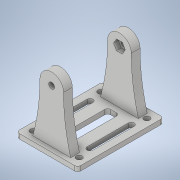
# Autodesk Inventor part: sideArmsHolder
Saved by Autodesk Inventor 2020 (Build 240168000, 168)
## iProperties
Created: 2019-05-25
Part Number: sideArmsHolder
Material: Generic
Document SubType Name: Modeling
Designer: Ryland Lillibridge
Density: 1 g/cm^3
Appearance: Default
Author: Ryland Lillibridge
Autodesk Inventor part; units mm, degrees
ref_plane "YZ Plane" through (0, 0, 0) normal (1, 0, 0) x (0, 1, 0)
ref_plane "XZ Plane" through (0, 0, 0) normal (0, 1, 0) x (-1, 0, 0)
ref_plane "XY Plane" through (0, 0, 0) normal (0, 0, 1) x (1, 0, 0)
sketch "Sketch1" plane through (0, 0, 0) normal (0, 1, 0) x (-1, 0, 0)
  circle A0 centre (0, 0) radius 31.75
  circle A1 centre (0, 0) radius 12.3825
  dimension "d0" = 63.5
  dimension "d1" = 24.765
  constraints: 2 centre point, 2 coincident
  measures "d0" diameter of A0
  measures "d1" diameter of A1
extrude "Extrusion1" add sketch "Sketch1" along normal blind 3.175 contours A0 | A1
sketch "Sketch2" plane through (0, 0, 0) normal (0, -1, 0) x (1, 0, 0)
  line L0 (1.524, 31.713403) -> (1.524, 0)
  line L1 (-1.524, 0) -> (-1.524, 31.713403)
  line L2 (-1.524, 35.89292) -> (0, 0) construction
  line L3 (1.524, 35.89292) -> (0, 0) construction
  line L4 (-1.524, 0) -> (1.524, 0)
  circle A0 centre (0, 0) radius 31.75
  dimension "d23" = 3.048
  constraints: 10 end point, 2 point on circle, 2 point on line, 1 parallel
  measures "d23" distance between parallel lines of L0 L1
extrude "Extrusion2" add sketch "Sketch2" along normal blind 1.524 contours L0 L4 L1 A0 picked at (0.169391, 10.581978)
pattern_circular "Circular Pattern1" count 8 over 360 about axis through (0, -10, 0) along (0, 1, 0) of "Extrusion2"
sketch "Sketch3" plane through (0, 0, 0) normal (0, -1, 0) x (1, 0, 0)
  circle A0 centre (0, 0) radius 12.573
  dimension "d11" = 25.146
  constraints: 1 centre point, 1 coincident
  measures "d11" diameter of A0
extrude "Extrusion3" add sketch "Sketch3" along normal blind 1.524
fillet "Fillet1" radius 0.635 16 edges at (1.524, -1.524, 22.0968) (-1.524, -1.524, 22.0968) (14.5472, -1.524, 16.7025) (16.7025, -1.524, 14.5472) (22.0968, -1.524, 1.524) (22.0968, -1.524, -1.524) (16.7025, -1.524, -14.5472) (14.5472, -1.524, -16.7025) (1.524, -1.524, -22.0968) (-1.524, -1.524, -22.0968) (-14.5472, -1.524, -16.7025) (-16.7025, -1.524, -14.5472) (-22.0968, -1.524, -1.524) (-22.0968, -1.524, 1.524) (-16.7025, -1.524, 14.5472) (-14.5472, -1.524, 16.7025)
sketch "Sketch4" plane through (0, 0, 0) normal (0, -1, 0) x (1, 0, 0)
  line L0 (0, 0) -> (25.813194, -10.692175)
  line L1 (0, 0) -> (27.94, 0) construction
  circle A0 centre (25.813194, -10.692175) radius 1.5875
  dimension "d15" = 27.94
  dimension "d16" = 22.5
  dimension "d17" = 3.175
  constraints: 4 end point, 1 centre point, 1 coincident, 1 equal length, 1 horizontal
  measures "d15" distance of L0.start L0.end
  measures "d16" angle of L0 L1
  measures "d17" diameter of A0
extrude "Extrusion4" cut sketch "Sketch4" against normal blind 25.4
pattern_circular "Circular Pattern2" count 8 over 360 about axis through (0, -10, 0) along (0, 1, 0) of "Extrusion4"
sketch "Sketch6" plane through (0, 0, 0) normal (0, 0, 1) x (1, 0, 0)
  line L0 (31.75, 3.175) -> (-31.75, 3.175)
  line L1 (0, 3.175) -> (19.05, 3.175)
  line L2 (19.05, 3.175) -> (-19.05, 3.175)
  line L3 (-19.05, 3.175) -> (-19.05, 53.975) construction
  line L4 (-19.05, 53.975) -> (19.05, 53.975) construction
  line L5 (19.05, 53.975) -> (19.05, 3.175) construction
  circle A0 centre (0, 53.975) radius 6.35
  arc A1 (6.35, 53.975) -> (19.05, 3.175) centre (114.3, 53.975) ccw
  line L6 (6.35, 53.975) -> (6.35, 55.853529) construction
  line L7 (-6.35, 53.975) -> (-6.35, 55.659663) construction
  arc A2 (-19.05, 3.175) -> (-6.35, 53.975) centre (-114.3, 53.975) ccw
  circle A3 centre (0, 53.975) radius 1.5875
  point P0 (0, 0)
  dimension "d28" = 19.05
  dimension "d29" = 38.1
  dimension "d30" = 50.8
  dimension "d31" = 12.7
  dimension "d32" = 3.175
  constraints: 14 end point, 6 point on circle, 4 centre point, 4 tangent, 3 point on line, 2 midpoint, 2 parallel, 2 perpendicular, 1 coincident, 1 horizontal, 1 vertical
  measures "d28" distance of L1.start L1.end
  measures "d29" distance of L3.end L4.end
  measures "d30" distance of L2.end L3.end
  measures "d31" diameter of A0
  measures "d32" diameter of A3
extrude "Extrusion6" add sketch "Sketch6" along normal mid plane 41.275
sketch "Sketch7" plane through (0, 3.175, 0) normal (0, 1, 0) x (1, 0, 0)
  line L0 (25.4, -15.875) -> (-25.4, -15.875)
  line L1 (-25.4, -15.875) -> (-25.4, 15.875)
  line L2 (-25.4, 15.875) -> (25.4, 15.875)
  line L3 (25.4, 15.875) -> (25.4, -15.875)
  line L4 (25.4, -15.875) -> (-25.4, 15.875) construction
  line L5 (-25.4, -15.875) -> (25.4, 15.875) construction
  point P0 (0, 0)
  dimension "d35" = 50.8
  dimension "d36" = 31.75
  constraints: 12 end point, 2 midpoint, 2 parallel, 1 horizontal, 1 perpendicular
  measures "d35" distance of L1.end L2.end
  measures "d36" distance of L0.end L1.end
extrude "Extrusion7" cut sketch "Sketch7" along normal blind 63.5
sketch "Sketch10" plane through (0, 3.175, 0) normal (0, 1, 0) x (1, 0, 0)
  line L0 (19.05, -38.1) -> (-19.05, -38.1)
  line L1 (-19.05, -38.1) -> (-19.05, 38.1)
  line L2 (-19.05, 38.1) -> (19.05, 38.1)
  line L3 (19.05, 38.1) -> (19.05, -38.1)
  line L4 (19.05, -38.1) -> (-19.05, 38.1) construction
  line L5 (-19.05, -38.1) -> (19.05, 38.1) construction
  line L6 (-19.05, -38.1) -> (-31.75, -38.1)
  line L7 (-31.75, -38.1) -> (-31.75, 38.1)
  line L8 (-31.75, 38.1) -> (-19.05, 38.1)
  line L9 (-19.05, 38.1) -> (-19.05, -38.1)
  line L10 (19.05, 38.1) -> (31.75, 38.1)
  line L11 (31.75, 38.1) -> (31.75, -38.1)
  line L12 (31.75, -38.1) -> (19.05, -38.1)
  line L13 (19.05, -38.1) -> (19.05, 38.1)
  point P0 (0, 0)
  dimension "d50" = 38.1
  dimension "d51" = 76.2
  dimension "d52" = 12.7
  dimension "d53" = 12.7
  constraints: 28 end point, 6 parallel, 3 horizontal, 3 perpendicular, 2 midpoint, 1 point on line
  measures "d50" distance of L1.end L2.end
  measures "d51" distance of L0.end L1.end
  measures "d52" distance of L7.end L8.end
  measures "d53" distance of L11.end L12.end
extrude "Extrusion9" cut sketch "Sketch10" against normal blind 63.5 contours L3 L10 L11 L12 | L6 L7 L8 L1
fillet "Fillet3" radius 6.35 4 edges at (19.05, 1.5875, 25.4) (19.05, 1.5875, -25.4) (-19.05, 1.5875, 25.4) (-19.05, 1.5875, -25.4)
sketch "Sketch11" plane through (0, 53.975, 15.875) normal (0, 0, -1) x (-1, 0, 0)
  arc A0 (6.35, 0) -> (-6.35, 0) centre (0, 0) ccw
  line L0 (1.587713, 2.75) -> (3.175426, 0)
  line L1 (3.175426, 0) -> (1.587713, -2.75)
  line L2 (1.587713, -2.75) -> (-1.587713, -2.75)
  line L3 (-1.587713, -2.75) -> (-3.175426, 0)
  line L4 (-3.175426, 0) -> (-1.587713, 2.75)
  line L5 (-1.587713, 2.75) -> (1.587713, 2.75)
  point P0 (0, -53.975)
  point P1 (0, 0)
  dimension "d57" = 5.5
  constraints: 12 end point, 1 coincident, 13 other
  measures "d57" distance between parallel lines of L5 L2
extrude "Extrusion10" cut sketch "Sketch11" against normal blind 2.54
mirror "Mirror1" about plane through (0, 0, 0) normal (0, 0, 1) of "Extrusion10"
fillet "Fillet4" radius 1.5875 2 edges at (0, 3.175, 20.6375) (0, 3.175, -20.6375)
chamfer "Chamfer3" [suppressed]
chamfer "Chamfer4" [suppressed]
sketch "Sketch12" plane through (0, 3.175, 0) normal (0, 1, 0) x (1, 0, 0)
  line L0 (9.380781, 15.875) -> (-9.380781, 15.875)
  line L1 (-3.175, -15.875) -> (3.175, -15.875)
  line L2 (3.175, -15.875) -> (3.175, 15.875)
  line L3 (3.175, 15.875) -> (-3.175, 15.875)
  line L4 (-3.175, 15.875) -> (-3.175, -15.875)
  line L5 (-3.175, -15.875) -> (3.175, 15.875) construction
  line L6 (3.175, -15.875) -> (-3.175, 15.875) construction
  line L7 (19.05, 21.997045) -> (19.05, -21.997045)
  line L8 (3.175, 15.875) -> (19.05, 15.875)
  line L9 (19.05, 15.875) -> (19.05, -15.875)
  line L10 (19.05, -15.875) -> (3.175, -15.875)
  line L11 (3.175, -15.875) -> (3.175, 15.875)
  line L12 (-19.05, 1.524) -> (-19.05, 16.894739)
  line L13 (-3.175, -15.875) -> (-19.05, -15.875)
  line L14 (-19.05, -15.875) -> (-19.05, 15.875)
  line L15 (-19.05, 15.875) -> (-3.175, 15.875)
  line L16 (-3.175, 15.875) -> (-3.175, -15.875)
  point P0 (0, 0)
  point P1 (19.05, -9.525)
  dimension "d67" = 6.35
  dimension "d73" = 31.75
  constraints: 28 end point, 6 parallel, 4 point on line, 3 horizontal, 3 perpendicular, 2 midpoint
  measures "d67" distance of L3.end L2.end
  measures "d73" distance of L8.end L9.end
fillet "Fillet5" [suppressed]
fillet "Fillet6" [suppressed]
fillet "Fillet7" [suppressed]
extrude "Extrusion12" [suppressed]
sketch "Sketch13" plane through (0, 0, 0) normal (0, 1, 0) x (-1, 0, 0)
  line L0 (28.089507, -35.463001) -> (-27.949059, -35.463001)
  line L1 (-27.949059, -35.463001) -> (-27.949059, 35.463001)
  line L2 (-27.949059, 35.463001) -> (28.089507, 35.463001)
  line L3 (28.089507, 35.463001) -> (28.089507, -35.463001)
  point P0 (0, 0)
  constraints: 8 end point, 2 parallel, 1 horizontal, 1 perpendicular
extrude "Extrusion13" cut sketch "Sketch13" along normal mid plane 50.8
sketch "Sketch14" plane through (0, 25.4, 0) normal (0, -1, 0) x (1, 0, 0)
  line L0 (10.200663, -20.6375) -> (-10.200663, -20.6375)
  line L1 (-10.200663, -20.6375) -> (14.645663, -20.6375)
  line L2 (14.645663, -20.6375) -> (14.645663, -15.875)
  line L3 (14.645663, -15.875) -> (-10.200663, -15.875)
  line L4 (-10.200663, -15.875) -> (-10.200663, -20.6375)
  line L5 (10.200663, 20.6375) -> (10.200663, -20.6375)
  line L6 (14.645663, -15.875) -> (-14.645663, -15.875)
  line L7 (-14.645663, -15.875) -> (-14.645663, -20.6375)
  line L8 (-14.645663, -20.6375) -> (14.645663, -20.6375)
  line L9 (14.645663, -20.6375) -> (14.645663, -15.875)
  line L10 (0, 0) -> (9.008264, 0)
  line L11 (-10.200663, 20.6375) -> (14.645663, 20.6375)
  line L12 (14.645663, 20.6375) -> (14.645663, 15.875)
  line L13 (14.645663, 15.875) -> (-10.200663, 15.875)
  line L14 (14.645663, 15.875) -> (-14.645663, 15.875)
  line L15 (-14.645663, 15.875) -> (-14.645663, 20.6375)
  line L16 (-14.645663, 20.6375) -> (14.645663, 20.6375)
  line L17 (10.200663, -20.6375) -> (14.645663, -15.875)
  line L18 (14.645663, -20.6375) -> (10.200663, -15.875)
  circle A0 centre (12.423163, -18.25625) radius 1.5875
  line L19 (0, -15.875) -> (0, -20.6375)
  line L20 (1.5875, -20.6375) -> (-1.5875, -20.6375)
  circle A1 centre (-12.423163, -18.25625) radius 1.5875
  circle A2 centre (12.423163, 18.25625) radius 1.5875
  circle A3 centre (-12.423163, 18.25625) radius 1.5875
  point P0 (-10.200663, -15.875)
  point P1 (-10.200663, 15.875)
  dimension "d78" = 4.445
  dimension "d79" = 4.445
  dimension "d82" = 3.175
  constraints: 36 end point, 10 symmetric about line, 4 centre point, 4 parallel, 3 horizontal, 3 midpoint, 2 perpendicular, 3 other
  measures "d78" distance between parallel lines of L2 L5
  measures "d79" distance between parallel lines of L7 L4
  measures "d82" diameter of A0
extrude "Extrusion14" add sketch "Sketch14" along normal blind 2.54 contours L17 A0 L18 L1 | L0 L19 L3 L5 | L5 L18 A0 L17 | L18 A0 L17 L2 | L3 L17 A0 L18 | L0 L4 L3 L19 | L4 L8 L7 L6 | L11 L12 L13 L5 | L5 L13 L14 L15 L16 L11
sketch "Sketch15" plane through (0, 53.975, -15.875) normal (0, 0, 1) x (1, 0, 0)
  line L0 (-14.645663, -28.575) -> (-14.645663, -31.115)
  line L1 (-14.645663, -28.575) -> (14.645663, -28.575)
  line L2 (14.645663, -28.575) -> (14.645663, -31.115)
  line L3 (14.645663, -31.115) -> (-14.645663, -31.115)
  line L4 (-14.645663, -31.115) -> (-14.645663, -28.575)
  point P0 (0, -53.975)
  constraints: 8 end point, 2 parallel, 1 horizontal, 1 perpendicular
extrude "Extrusion15" add sketch "Sketch15" along normal blind 32.258
sketch "Sketch17" plane through (0, 25.4, 0) normal (0, 1, 0) x (1, 0, 0)
  line L0 (0, 12.7) -> (-12.7, 12.7)
  line L1 (-12.7, 12.7) -> (-12.7, -12.7)
  line L2 (-12.7, -12.7) -> (12.7, -12.7)
  line L3 (12.7, -12.7) -> (12.7, 12.7)
  line L4 (12.7, 12.7) -> (0, 12.7)
  line L5 (12.7, 12.7) -> (9.525, 12.7)
  line L6 (9.525, 12.7) -> (9.525, -12.7)
  line L7 (9.525, -12.7) -> (12.7, -12.7)
  line L8 (12.7, -12.7) -> (12.7, 12.7)
  line L9 (-12.7, 12.7) -> (-9.525, 12.7)
  line L10 (-9.525, -12.7) -> (-12.7, -12.7)
  line L11 (-12.7, -12.7) -> (-12.7, 12.7)
  line L12 (-1.587713, 12.7) -> (1.587713, 12.7)
  line L13 (1.587713, -12.7) -> (-1.587713, -12.7)
  line L14 (-6.35, 12.7) -> (-3.175, 12.7)
  line L15 (-3.175, -12.7) -> (-6.35, -12.7)
  line L16 (6.35, 12.7) -> (6.35, -12.7)
  line L17 (9.525, -12.7) -> (9.525, 12.7)
  line L18 (9.525, 12.7) -> (-3.175, 12.7)
  line L19 (6.35, -12.7) -> (9.525, -12.7)
  line L20 (3.175, 12.7) -> (3.175, -12.7)
  line L21 (6.35, -12.7) -> (6.35, 12.7)
  line L22 (6.35, 12.7) -> (-6.35, 12.7)
  line L23 (3.175, -12.7) -> (6.35, -12.7)
  line L24 (0, 12.7) -> (0, -12.7)
  line L25 (3.175, -12.7) -> (3.175, 12.7)
  line L26 (3.175, 12.7) -> (-9.525, 12.7)
  line L27 (0, -12.7) -> (3.175, -12.7)
  line L28 (-3.175, 12.7) -> (-3.175, -12.7)
  line L29 (0, -12.7) -> (0, 12.7)
  line L30 (0, 12.7) -> (-12.7, 12.7)
  line L31 (-3.175, -12.7) -> (0, -12.7)
  line L32 (-6.35, 12.7) -> (-6.35, -12.7)
  line L33 (-3.175, -12.7) -> (-3.175, 12.7)
  line L34 (-3.175, 12.7) -> (-15.875, 12.7)
  line L35 (-6.35, -12.7) -> (-3.175, -12.7)
  line L36 (-9.525, 12.7) -> (-9.525, -12.7)
  line L37 (-6.35, -12.7) -> (-6.35, 12.7)
  line L38 (-6.35, 12.7) -> (-19.05, 12.7)
  line L39 (-9.525, -12.7) -> (-6.35, -12.7)
  line L40 (-12.7, 12.7) -> (-12.7, -12.7)
  line L41 (-9.525, -12.7) -> (-9.525, 12.7)
  line L42 (-9.525, 12.7) -> (-22.225, 12.7)
  line L43 (-12.7, -12.7) -> (-9.525, -12.7)
  point P0 (0, 0)
  point P1 (3.175, -12.7)
  dimension "d94" = 12.7
  dimension "d95" = 25.4
  dimension "d96" = 25.4
  dimension "d97" = 3.175
  dimension "d98" = 3.175
  dimension "d99" = 3.175
  dimension "d102" = 3.175
  constraints: 88 end point, 6 equal length, 6 point on line, 5 horizontal, 4 perpendicular, 1 collinear, 1 midpoint, 69 other
  measures "d94" distance of L0.start L0.end
  measures "d95" distance of L0.end L1.end
  measures "d96" distance of L1.end L2.end
  measures "d97" distance of L7.end L6.end
  measures "d98" distance of L10.start L10.end
  measures "d99" distance of L15.start L15.end
  measures "d102" distance of L5.end L16.start
extrude "Extrusion17" cut sketch "Sketch17" against normal blind 32.258 contours L24 L2 L28 L0 | L4 L20 L2 L24 | L36 L2 L1 L0 | L4 L3 L2 L6
sketch "Sketch18" plane through (14.645663, 22.86, 20.6375) normal (1, 0, 0) x (0, 0, -1)
  line L0 (0, 2.54) -> (41.275, 2.54) projected
  line L1 (0, 2.54) -> (41.275, 2.54)
  line L2 (41.275, 2.54) -> (41.275, 0)
  line L3 (41.275, 0) -> (0, 0)
  line L4 (0, 0) -> (0, 2.54)
  point P0 (20.6375, -22.86)
  constraints: 8 end point, 2 parallel, 1 horizontal, 1 perpendicular
extrude "Extrusion18" add sketch "Sketch18" along normal blind 1.905
mirror "Mirror2" about plane through (0, 0, 0) normal (1, 0, 0) of "Extrusion18"
sketch "Sketch20" plane through (0, 0, 20.6375) normal (0, 0, 1) x (1, 0, 0)
  line L0 (-16.550663, 25.4) -> (-16.550663, 22.86)
  line L1 (16.550663, 22.86) -> (16.550663, 25.4)
  line L2 (-16.550663, 25.4) -> (16.550663, 25.4)
  line L3 (16.550663, 25.4) -> (16.550663, 22.86)
  line L4 (16.550663, 22.86) -> (-16.550663, 22.86)
  line L5 (-16.550663, 22.86) -> (-16.550663, 25.4)
  point P0 (0, 0)
  constraints: 8 end point, 2 parallel, 1 horizontal, 1 perpendicular
extrude "Extrusion19" add sketch "Sketch20" along normal blind 2.54
mirror "Mirror3" about plane through (0, 0, 0) normal (0, 0, 1) of "Extrusion19"
fillet "Fillet8" radius 1.5875 16 edges at (16.5507, 24.13, 23.1775) (-16.5507, 24.13, 23.1775) (-9.525, 24.13, -12.7) (3.175, 24.13, -12.7) (12.7, 24.13, -12.7) (-16.5507, 24.13, -23.1775) (9.525, 24.13, -12.7) (-3.175, 24.13, -12.7) (-12.7, 24.13, -12.7) (-3.175, 24.13, 12.7) (-12.7, 24.13, 12.7) (16.5507, 24.13, -23.1775) (12.7, 24.13, 12.7) (3.175, 24.13, 12.7) (-9.525, 24.13, 12.7) (9.525, 24.13, 12.7)
body "Solid1"
